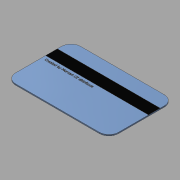
# Autodesk Inventor part: card
Saved by Autodesk Inventor 2014 SP2 (Build 180246200, 246)
## iProperties
Created: 2016-01-21
Part Number: card
Material: ABS plast
Document SubType Name: Modeling
Designer: Mervart
Mass: 4.83646 g
Surface Area: 97.3494 cm^2
Volume: 4.56269 cm^3
Density: 1.06 g/cm^3
Appearance: Hladká – bílá
LastSaveDate: 21.09.2010
Hmotnost: 0
Author: Mervart
Autodesk Inventor part; units mm, degrees
(part 1 of 2)
ref_plane "YZ Plane" through (0, 0, 0) normal (1, 0, 0) x (0, 1, 0)
sketch "Náčrt4" plane through (0, 0, 0) normal (0, 0, 1) x (1, 0, 0)
  line L0 (-42.75, -27) -> (42.75, -27)
  line L1 (42.75, -27) -> (42.75, 27)
  line L2 (42.75, 27) -> (-42.75, 27)
  line L3 (-42.75, 27) -> (-42.75, -27)
  line L4 (-42.75, -27) -> (42.75, 27) construction
  line L5 (42.75, -27) -> (-42.75, 27) construction
  point P0 (0, 0)
  dimension "d0" = 85.5
  dimension "d1" = 54
  constraints: 12 end point, 2 midpoint, 2 parallel, 1 horizontal, 1 perpendicular
  measures "d0" distance of L2.end L1.end
  measures "d1" distance of L2.end L0.start
extrude "Vysunutí1" add sketch "Náčrt4" along normal blind 1
fillet "Zaoblení1" radius 8 4 edges at (42.75, -27, 0.5) (42.75, 27, 0.5) (-42.75, 27, 0.5) (-42.75, -27, 0.5)
sketch "Náčrt5" plane through (0, 0, 1) normal (0, 0, 1) x (1, 0, 0)
  arc A0 (-42.75, -19) -> (-34.75, -27) centre (-34.75, -19) ccw construction
  line L0 (-34.75, -27) -> (34.75, -27) construction
  arc A1 (34.75, -27) -> (42.75, -19) centre (34.75, -19) ccw construction
  line L1 (42.75, -19) -> (42.75, 19) construction
  arc A2 (42.75, 19) -> (34.75, 27) centre (34.75, 19) ccw construction
  line L2 (34.75, 27) -> (-34.75, 27) construction
  arc A3 (-34.75, 27) -> (-42.75, 19) centre (-34.75, 19) ccw construction
  line L3 (-42.75, 19) -> (-42.75, -19) construction
  line L4 (42.75, 15.5948) -> (-42.75, 15.5948)
  line L5 (42.75, 5.8734) -> (-42.75, 5.8734)
  line L6 (-42.75, 5.8734) -> (-42.75, 15.5948)
  line L7 (42.75, 5.8734) -> (42.75, 15.5948)
  point P0 (0, 0)
  constraints: 8 end point, 4 point on line, 2 collinear, 2 perpendicular
ref_plane "Pracovní rovina1" through (42.75, 5.8734, 1) normal (0, 1, 0) x (-1, 0, 0)
ref_plane "Pracovní rovina2" through (42.75, 15.5948, 1) normal (0, 1, 0) x (-1, 0, 0)
split body "Rozdělit1" result two bodies by plane through (42.75, 15.5948, 1) normal (0, 1, 0) first body at (-11.5833, 19.3965, 0.5)
split body "Rozdělit2" result two bodies by plane through (42.75, 5.8734, 1) normal (0, 1, 0) bodies 3 first body at (-14.25, 12.3543, 0.5)
sketch "Náčrt6" plane through (0, 0, 1) normal (0, 0, 1) x (1, 0, 0)
  line L0 (-40.2387, 4.1503) -> (29.6053, 4.1503) construction
  line L1 (29.6053, 4.1503) -> (29.6053, -0.4729) construction
  line L2 (29.6053, -0.4729) -> (-40.2387, -0.4729) construction
  line L3 (-40.2387, -0.4729) -> (-40.2387, 4.1503) construction
  spline S0 degree 2 poles (-39.2549, 2.0255) (-39.4494, 2.0255) (-39.7784, 2.1567) (-39.8983, 2.288) knots 0 0 0 1 2 2 2
  spline S1 degree 2 poles (-39.8983, 2.288) (-40.0183, 2.4177) (-40.1496, 2.8067) (-40.1496, 3.0595) knots 0 0 0 1 2 2 2
  spline S2 degree 2 poles (-40.1496, 3.0595) (-40.1496, 3.3107) (-40.0215, 3.6835) (-39.9, 3.8213) knots 0 0 0 1 2 2 2
  spline S3 degree 2 poles (-39.9, 3.8213) (-39.78, 3.9558) (-39.4526, 4.0968) (-39.2501, 4.0968) knots 0 0 0 1 2 2 2
  spline S4 degree 2 poles (-39.2501, 4.0968) (-39.1496, 4.0968) (-38.9729, 4.0676) (-38.8983, 4.0449) knots 0 0 0 1 2 2 2
  spline S5 degree 2 poles (-38.8983, 4.0449) (-38.8335, 4.0238) (-38.699, 3.9639) (-38.6325, 3.9282) knots 0 0 0 1 2 2 2
  line L4 (-38.6325, 3.9282) -> (-38.6325, 3.6073)
  line L5 (-38.6325, 3.6073) -> (-38.6536, 3.6073)
  spline S6 degree 2 poles (-38.6536, 3.6073) (-38.6893, 3.6397) (-38.7995, 3.7305) (-38.8789, 3.7742) knots 0 0 0 1 2 2 2
  spline S7 degree 2 poles (-38.8789, 3.7742) (-38.9551, 3.8164) (-39.135, 3.8699) (-39.2517, 3.8699) knots 0 0 0 1 2 2 2
  spline S8 degree 2 poles (-39.2517, 3.8699) (-39.3797, 3.8699) (-39.6082, 3.7645) (-39.6941, 3.664) knots 0 0 0 1 2 2 2
  spline S9 degree 2 poles (-39.6941, 3.664) (-39.7784, 3.5619) (-39.8724, 3.2524) (-39.8724, 3.0595) knots 0 0 0 1 2 2 2
  spline S10 degree 2 poles (-39.8724, 3.0595) (-39.8724, 2.8537) (-39.7736, 2.5571) (-39.6877, 2.455) knots 0 0 0 1 2 2 2
  spline S11 degree 2 poles (-39.6877, 2.455) (-39.6034, 2.3561) (-39.3781, 2.2556) (-39.2517, 2.2556) knots 0 0 0 1 2 2 2
  spline S12 degree 2 poles (-39.2517, 2.2556) (-39.1366, 2.2556) (-38.9405, 2.3123) (-38.8643, 2.3545) knots 0 0 0 1 2 2 2
  spline S13 degree 2 poles (-38.8643, 2.3545) (-38.7914, 2.3966) (-38.6828, 2.4841) (-38.652, 2.5149) knots 0 0 0 1 2 2 2
  line L6 (-38.652, 2.5149) -> (-38.6325, 2.5149)
  line L7 (-38.6325, 2.5149) -> (-38.6325, 2.1973)
  spline S14 degree 2 poles (-38.6325, 2.1973) (-38.699, 2.1665) (-38.8157, 2.1097) (-38.8983, 2.0838) knots 0 0 0 1 2 2 2
  spline S15 degree 2 poles (-38.8983, 2.0838) (-38.9859, 2.0546) (-39.135, 2.0255) (-39.2549, 2.0255) knots 0 0 0 1 2 2 2
  line L8 (-37.6082, 3.2913) -> (-37.6212, 3.2913)
  spline S16 degree 2 poles (-37.6212, 3.2913) (-37.6504, 3.2994) (-37.7136, 3.3026) (-37.7573, 3.3026) knots 0 0 0 1 2 2 2
  spline S17 degree 2 poles (-37.7573, 3.3026) (-37.8595, 3.3026) (-38.0604, 3.2135) (-38.1512, 3.126) knots 0 0 0 1 2 2 2
  line L9 (-38.1512, 3.126) -> (-38.1512, 2.0611)
  line L10 (-38.1512, 2.0611) -> (-38.404, 2.0611)
  line L11 (-38.404, 2.0611) -> (-38.404, 3.5619)
  line L12 (-38.404, 3.5619) -> (-38.1512, 3.5619)
  line L13 (-38.1512, 3.5619) -> (-38.1512, 3.3383)
  spline S18 degree 2 poles (-38.1512, 3.3383) (-38.0134, 3.4614) (-37.8076, 3.5619) (-37.7103, 3.5619) knots 0 0 0 1 2 2 2
  spline S19 degree 2 poles (-37.7103, 3.5619) (-37.6714, 3.5619) (-37.6325, 3.5587) (-37.6082, 3.5538) knots 0 0 0 1 2 2 2
  line L14 (-37.6082, 3.5538) -> (-37.6082, 3.2913)
  spline S20 degree 2 poles (-36.7606, 2.0271) (-37.1204, 2.0271) (-37.5159, 2.4307) (-37.5159, 2.8034) knots 0 0 0 1 2 2 2
  spline S21 degree 2 poles (-37.5159, 2.8034) (-37.5159, 3.1697) (-37.1317, 3.6041) (-36.8222, 3.6041) knots 0 0 0 1 2 2 2
  spline S22 degree 2 poles (-36.8222, 3.6041) (-36.6828, 3.6041) (-36.4672, 3.523) (-36.3878, 3.4371) knots 0 0 0 1 2 2 2
  spline S23 degree 2 poles (-36.3878, 3.4371) (-36.3068, 3.3512) (-36.2209, 3.1033) (-36.2209, 2.9234) knots 0 0 0 1 2 2 2
  line L15 (-36.2209, 2.9234) -> (-36.2209, 2.7856)
  line L16 (-36.2209, 2.7856) -> (-37.2598, 2.7856)
  spline S24 degree 2 poles (-37.2598, 2.7856) (-37.2598, 2.5247) (-36.9972, 2.2475) (-36.7638, 2.2475) knots 0 0 0 1 2 2 2
  spline S25 degree 2 poles (-36.7638, 2.2475) (-36.6812, 2.2475) (-36.5207, 2.2848) (-36.4559, 2.314) knots 0 0 0 1 2 2 2
  spline S26 degree 2 poles (-36.4559, 2.314) (-36.3878, 2.3464) (-36.2938, 2.4031) (-36.263, 2.429) knots 0 0 0 1 2 2 2
  line L17 (-36.263, 2.429) -> (-36.2484, 2.429)
  line L18 (-36.2484, 2.429) -> (-36.2484, 2.1535)
  spline S27 degree 2 poles (-36.2484, 2.1535) (-36.2922, 2.1357) (-36.4251, 2.0838) (-36.477, 2.0692) knots 0 0 0 1 2 2 2
  spline S28 degree 2 poles (-36.477, 2.0692) (-36.5499, 2.0482) (-36.6698, 2.0271) (-36.7606, 2.0271) knots 0 0 0 1 2 2 2
  spline S29 degree 2 poles (-36.4672, 2.9785) (-36.4705, 3.0806) (-36.5126, 3.2297) (-36.5531, 3.2799) knots 0 0 0 1 2 2 2
  spline S30 degree 2 poles (-36.5531, 3.2799) (-36.5969, 3.3366) (-36.7347, 3.3966) (-36.8368, 3.3966) knots 0 0 0 1 2 2 2
  spline S31 degree 2 poles (-36.8368, 3.3966) (-36.9372, 3.3966) (-37.0783, 3.3366) (-37.1366, 3.2783) knots 0 0 0 1 2 2 2
  spline S32 degree 2 poles (-37.1366, 3.2783) (-37.1933, 3.2183) (-37.2517, 3.0741) (-37.2598, 2.9785) knots 0 0 0 1 2 2 2
  line L19 (-37.2598, 2.9785) -> (-36.4672, 2.9785)
  spline S33 degree 2 poles (-35.1285, 2.22) (-35.1593, 2.1973) (-35.263, 2.1162) (-35.3116, 2.0919) knots 0 0 0 1 2 2 2
  spline S34 degree 2 poles (-35.3116, 2.0919) (-35.3781, 2.0563) (-35.5029, 2.019) (-35.6163, 2.019) knots 0 0 0 1 2 2 2
  spline S35 degree 2 poles (-35.6163, 2.019) (-35.7087, 2.019) (-35.8757, 2.0887) (-35.9389, 2.1519) knots 0 0 0 1 2 2 2
  spline S36 degree 2 poles (-35.9389, 2.1519) (-35.9988, 2.2135) (-36.0718, 2.395) (-36.0718, 2.4955) knots 0 0 0 1 2 2 2
  spline S37 degree 2 poles (-36.0718, 2.4955) (-36.0718, 2.6511) (-35.9405, 2.8715) (-35.7979, 2.9347) knots 0 0 0 1 2 2 2
  spline S38 degree 2 poles (-35.7979, 2.9347) (-35.6714, 2.9931) (-35.3278, 3.0368) (-35.1285, 3.0482) knots 0 0 0 1 2 2 2
  line L20 (-35.1285, 3.0482) -> (-35.1285, 3.0968)
  spline S39 degree 2 poles (-35.1285, 3.0968) (-35.1285, 3.1843) (-35.182, 3.2929) (-35.2306, 3.3237) knots 0 0 0 1 2 2 2
  spline S40 degree 2 poles (-35.2306, 3.3237) (-35.2792, 3.3545) (-35.4186, 3.3739) (-35.4932, 3.3739) knots 0 0 0 1 2 2 2
  spline S41 degree 2 poles (-35.4932, 3.3739) (-35.5807, 3.3739) (-35.8173, 3.3221) (-35.9356, 3.2718) knots 0 0 0 1 2 2 2
  line L21 (-35.9356, 3.2718) -> (-35.9502, 3.2718)
  line L22 (-35.9502, 3.2718) -> (-35.9502, 3.5295)
  spline S42 degree 2 poles (-35.9502, 3.5295) (-35.8805, 3.549) (-35.6196, 3.5976) (-35.4915, 3.5976) knots 0 0 0 1 2 2 2
  spline S43 degree 2 poles (-35.4915, 3.5976) (-35.336, 3.5976) (-35.1236, 3.549) (-35.0394, 3.4858) knots 0 0 0 1 2 2 2
  spline S44 degree 2 poles (-35.0394, 3.4858) (-34.9567, 3.4242) (-34.8757, 3.2281) (-34.8757, 3.0871) knots 0 0 0 1 2 2 2
  line L23 (-34.8757, 3.0871) -> (-34.8757, 2.0611)
  line L24 (-34.8757, 2.0611) -> (-35.1285, 2.0611)
  line L25 (-35.1285, 2.0611) -> (-35.1285, 2.22)
  line L26 (-35.1285, 2.4307) -> (-35.1285, 2.8472)
  spline S45 degree 2 poles (-35.1285, 2.8472) (-35.2193, 2.8391) (-35.4932, 2.8115) (-35.5791, 2.7856) knots 0 0 0 1 2 2 2
  spline S46 degree 2 poles (-35.5791, 2.7856) (-35.6795, 2.7548) (-35.8108, 2.6268) (-35.8108, 2.5133) knots 0 0 0 1 2 2 2
  spline S47 degree 2 poles (-35.8108, 2.5133) (-35.8108, 2.3837) (-35.665, 2.2524) (-35.5256, 2.2524) knots 0 0 0 1 2 2 2
  spline S48 degree 2 poles (-35.5256, 2.2524) (-35.4073, 2.2524) (-35.2128, 2.3545) (-35.1285, 2.4307) knots 0 0 0 1 2 2 2
  spline S49 degree 2 poles (-34.0669, 2.0319) (-34.2727, 2.0319) (-34.5045, 2.267) (-34.5045, 2.5214) knots 0 0 0 1 2 2 2
  line L27 (-34.5045, 2.5214) -> (-34.5045, 3.3529)
  line L28 (-34.5045, 3.3529) -> (-34.6747, 3.3529)
  line L29 (-34.6747, 3.3529) -> (-34.6747, 3.5619)
  line L30 (-34.6747, 3.5619) -> (-34.5045, 3.5619)
  line L31 (-34.5045, 3.5619) -> (-34.5045, 3.9931)
  line L32 (-34.5045, 3.9931) -> (-34.2517, 3.9931)
  line L33 (-34.2517, 3.9931) -> (-34.2517, 3.5619)
  line L34 (-34.2517, 3.5619) -> (-33.7865, 3.5619)
  line L35 (-33.7865, 3.5619) -> (-33.7865, 3.3529)
  line L36 (-33.7865, 3.3529) -> (-34.2517, 3.3529)
  line L37 (-34.2517, 3.3529) -> (-34.2517, 2.6381)
  spline S50 degree 2 poles (-34.2517, 2.6381) (-34.2517, 2.5247) (-34.2436, 2.3999) (-34.216, 2.3464) knots 0 0 0 1 2 2 2
  spline S51 degree 2 poles (-34.216, 2.3464) (-34.1933, 2.2994) (-34.0912, 2.2524) (-34.0037, 2.2524) knots 0 0 0 1 2 2 2
  spline S52 degree 2 poles (-34.0037, 2.2524) (-33.9421, 2.2524) (-33.827, 2.2896) (-33.8011, 2.301) knots 0 0 0 1 2 2 2
  line L38 (-33.8011, 2.301) -> (-33.7865, 2.301)
  line L39 (-33.7865, 2.301) -> (-33.7865, 2.0741)
  spline S53 degree 2 poles (-33.7865, 2.0741) (-33.8578, 2.0546) (-34.0037, 2.0319) (-34.0669, 2.0319) knots 0 0 0 1 2 2 2
  spline S54 degree 2 poles (-32.9486, 2.0271) (-33.3084, 2.0271) (-33.7039, 2.4307) (-33.7039, 2.8034) knots 0 0 0 1 2 2 2
  spline S55 degree 2 poles (-33.7039, 2.8034) (-33.7039, 3.1697) (-33.3197, 3.6041) (-33.0102, 3.6041) knots 0 0 0 1 2 2 2
  spline S56 degree 2 poles (-33.0102, 3.6041) (-32.8708, 3.6041) (-32.6552, 3.523) (-32.5758, 3.4371) knots 0 0 0 1 2 2 2
  spline S57 degree 2 poles (-32.5758, 3.4371) (-32.4948, 3.3512) (-32.4089, 3.1033) (-32.4089, 2.9234) knots 0 0 0 1 2 2 2
  line L40 (-32.4089, 2.9234) -> (-32.4089, 2.7856)
  line L41 (-32.4089, 2.7856) -> (-33.4478, 2.7856)
  spline S58 degree 2 poles (-33.4478, 2.7856) (-33.4478, 2.5247) (-33.1852, 2.2475) (-32.9518, 2.2475) knots 0 0 0 1 2 2 2
  spline S59 degree 2 poles (-32.9518, 2.2475) (-32.8692, 2.2475) (-32.7087, 2.2848) (-32.6439, 2.314) knots 0 0 0 1 2 2 2
  spline S60 degree 2 poles (-32.6439, 2.314) (-32.5758, 2.3464) (-32.4818, 2.4031) (-32.451, 2.429) knots 0 0 0 1 2 2 2
  line L42 (-32.451, 2.429) -> (-32.4364, 2.429)
  line L43 (-32.4364, 2.429) -> (-32.4364, 2.1535)
  spline S61 degree 2 poles (-32.4364, 2.1535) (-32.4802, 2.1357) (-32.6131, 2.0838) (-32.665, 2.0692) knots 0 0 0 1 2 2 2
  spline S62 degree 2 poles (-32.665, 2.0692) (-32.7379, 2.0482) (-32.8578, 2.0271) (-32.9486, 2.0271) knots 0 0 0 1 2 2 2
  spline S63 degree 2 poles (-32.6552, 2.9785) (-32.6585, 3.0806) (-32.7006, 3.2297) (-32.7411, 3.2799) knots 0 0 0 1 2 2 2
  spline S64 degree 2 poles (-32.7411, 3.2799) (-32.7849, 3.3366) (-32.9227, 3.3966) (-33.0248, 3.3966) knots 0 0 0 1 2 2 2
  spline S65 degree 2 poles (-33.0248, 3.3966) (-33.1253, 3.3966) (-33.2663, 3.3366) (-33.3246, 3.2783) knots 0 0 0 1 2 2 2
  spline S66 degree 2 poles (-33.3246, 3.2783) (-33.3813, 3.2183) (-33.4397, 3.0741) (-33.4478, 2.9785) knots 0 0 0 1 2 2 2
  line L44 (-33.4478, 2.9785) -> (-32.6552, 2.9785)
  line L45 (-30.9988, 2.0611) -> (-31.2517, 2.0611)
  line L46 (-31.2517, 2.0611) -> (-31.2517, 2.2135)
  spline S67 degree 2 poles (-31.2517, 2.2135) (-31.31, 2.1648) (-31.3959, 2.1) (-31.4543, 2.0725) knots 0 0 0 1 2 2 2
  spline S68 degree 2 poles (-31.4543, 2.0725) (-31.5077, 2.0465) (-31.6228, 2.019) (-31.699, 2.019) knots 0 0 0 1 2 2 2
  spline S69 degree 2 poles (-31.699, 2.019) (-31.8222, 2.019) (-32.0296, 2.1211) (-32.1026, 2.22) knots 0 0 0 1 2 2 2
  spline S70 degree 2 poles (-32.1026, 2.22) (-32.1755, 2.3188) (-32.2565, 2.6106) (-32.2565, 2.8002) knots 0 0 0 1 2 2 2
  spline S71 degree 2 poles (-32.2565, 2.8002) (-32.2565, 2.9979) (-32.1544, 3.2864) (-32.0653, 3.395) knots 0 0 0 1 2 2 2
  spline S72 degree 2 poles (-32.0653, 3.395) (-31.9826, 3.4922) (-31.7509, 3.6041) (-31.6228, 3.6041) knots 0 0 0 1 2 2 2
  spline S73 degree 2 poles (-31.6228, 3.6041) (-31.511, 3.6041) (-31.3441, 3.5538) (-31.2517, 3.502) knots 0 0 0 1 2 2 2
  line L47 (-31.2517, 3.502) -> (-31.2517, 4.1503)
  line L48 (-31.2517, 4.1503) -> (-30.9988, 4.1503)
  line L49 (-30.9988, 4.1503) -> (-30.9988, 2.0611)
  line L50 (-31.2517, 2.4258) -> (-31.2517, 3.2929)
  spline S74 degree 2 poles (-31.2517, 3.2929) (-31.3457, 3.3383) (-31.4948, 3.3723) (-31.5807, 3.3723) knots 0 0 0 1 2 2 2
  spline S75 degree 2 poles (-31.5807, 3.3723) (-31.7752, 3.3723) (-31.9956, 3.0806) (-31.9956, 2.805) knots 0 0 0 1 2 2 2
  spline S76 degree 2 poles (-31.9956, 2.805) (-31.9956, 2.5392) (-31.827, 2.2589) (-31.6407, 2.2589) knots 0 0 0 1 2 2 2
  spline S77 degree 2 poles (-31.6407, 2.2589) (-31.5418, 2.2589) (-31.3408, 2.3496) (-31.2517, 2.4258) knots 0 0 0 1 2 2 2
  spline S78 degree 2 poles (-28.5159, 2.8358) (-28.5159, 2.4679) (-28.8724, 2.019) (-29.1415, 2.019) knots 0 0 0 1 2 2 2
  spline S79 degree 2 poles (-29.1415, 2.019) (-29.263, 2.019) (-29.4364, 2.0789) (-29.5207, 2.1308) knots 0 0 0 1 2 2 2
  line L51 (-29.5207, 2.1308) -> (-29.5369, 2.0611)
  line L52 (-29.5369, 2.0611) -> (-29.7736, 2.0611)
  line L53 (-29.7736, 2.0611) -> (-29.7736, 4.1503)
  line L54 (-29.7736, 4.1503) -> (-29.5207, 4.1503)
  line L55 (-29.5207, 4.1503) -> (-29.5207, 3.4047)
  spline S80 degree 2 poles (-29.5207, 3.4047) (-29.4251, 3.4906) (-29.203, 3.6041) (-29.062, 3.6041) knots 0 0 0 1 2 2 2
  spline S81 degree 2 poles (-29.062, 3.6041) (-28.8076, 3.6041) (-28.5159, 3.1973) (-28.5159, 2.8358) knots 0 0 0 1 2 2 2
  spline S82 degree 2 poles (-28.7768, 2.8164) (-28.7768, 3.0854) (-28.9405, 3.3642) (-29.122, 3.3642) knots 0 0 0 1 2 2 2
  spline S83 degree 2 poles (-29.122, 3.3642) (-29.2241, 3.3642) (-29.4348, 3.267) (-29.5207, 3.1924) knots 0 0 0 1 2 2 2
  line L56 (-29.5207, 3.1924) -> (-29.5207, 2.3318)
  spline S84 degree 2 poles (-29.5207, 2.3318) (-29.4251, 2.2848) (-29.2776, 2.2459) (-29.1901, 2.2459) knots 0 0 0 1 2 2 2
  spline S85 degree 2 poles (-29.1901, 2.2459) (-28.9972, 2.2459) (-28.7768, 2.5198) (-28.7768, 2.8164) knots 0 0 0 1 2 2 2
  line L57 (-27.075, 3.5619) -> (-27.8821, 1.5084)
  line L58 (-27.8821, 1.5084) -> (-28.1528, 1.5084)
  line L59 (-28.1528, 1.5084) -> (-27.8838, 2.1341)
  line L60 (-27.8838, 2.1341) -> (-28.4283, 3.5619)
  line L61 (-28.4283, 3.5619) -> (-28.156, 3.5619)
  line L62 (-28.156, 3.5619) -> (-27.746, 2.4501)
  line L63 (-27.746, 2.4501) -> (-27.3376, 3.5619)
  line L64 (-27.3376, 3.5619) -> (-27.075, 3.5619)
  line L65 (-24.2906, 2.0611) -> (-24.5564, 2.0611)
  line L66 (-24.5564, 2.0611) -> (-24.5564, 3.784)
  line L67 (-24.5564, 3.784) -> (-25.0783, 2.6122)
  line L68 (-25.0783, 2.6122) -> (-25.2403, 2.6122)
  line L69 (-25.2403, 2.6122) -> (-25.7573, 3.784)
  line L70 (-25.7573, 3.784) -> (-25.7573, 2.0611)
  line L71 (-25.7573, 2.0611) -> (-26.0053, 2.0611)
  line L72 (-26.0053, 2.0611) -> (-26.0053, 4.0611)
  line L73 (-26.0053, 4.0611) -> (-25.6423, 4.0611)
  line L74 (-25.6423, 4.0611) -> (-25.1431, 2.9477)
  line L75 (-25.1431, 2.9477) -> (-24.6601, 4.0611)
  line L76 (-24.6601, 4.0611) -> (-24.2906, 4.0611)
  line L77 (-24.2906, 4.0611) -> (-24.2906, 2.0611)
  spline S86 degree 2 poles (-23.2533, 2.0271) (-23.6131, 2.0271) (-24.0086, 2.4307) (-24.0086, 2.8034) knots 0 0 0 1 2 2 2
  spline S87 degree 2 poles (-24.0086, 2.8034) (-24.0086, 3.1697) (-23.6244, 3.6041) (-23.3149, 3.6041) knots 0 0 0 1 2 2 2
  spline S88 degree 2 poles (-23.3149, 3.6041) (-23.1755, 3.6041) (-22.9599, 3.523) (-22.8805, 3.4371) knots 0 0 0 1 2 2 2
  spline S89 degree 2 poles (-22.8805, 3.4371) (-22.7995, 3.3512) (-22.7136, 3.1033) (-22.7136, 2.9234) knots 0 0 0 1 2 2 2
  line L78 (-22.7136, 2.9234) -> (-22.7136, 2.7856)
  line L79 (-22.7136, 2.7856) -> (-23.7525, 2.7856)
  spline S90 degree 2 poles (-23.7525, 2.7856) (-23.7525, 2.5247) (-23.4899, 2.2475) (-23.2565, 2.2475) knots 0 0 0 1 2 2 2
  spline S91 degree 2 poles (-23.2565, 2.2475) (-23.1739, 2.2475) (-23.0134, 2.2848) (-22.9486, 2.314) knots 0 0 0 1 2 2 2
  spline S92 degree 2 poles (-22.9486, 2.314) (-22.8805, 2.3464) (-22.7865, 2.4031) (-22.7557, 2.429) knots 0 0 0 1 2 2 2
  line L80 (-22.7557, 2.429) -> (-22.7411, 2.429)
  line L81 (-22.7411, 2.429) -> (-22.7411, 2.1535)
  spline S93 degree 2 poles (-22.7411, 2.1535) (-22.7849, 2.1357) (-22.9178, 2.0838) (-22.9697, 2.0692) knots 0 0 0 1 2 2 2
  spline S94 degree 2 poles (-22.9697, 2.0692) (-23.0426, 2.0482) (-23.1625, 2.0271) (-23.2533, 2.0271) knots 0 0 0 1 2 2 2
  spline S95 degree 2 poles (-22.9599, 2.9785) (-22.9632, 3.0806) (-23.0053, 3.2297) (-23.0458, 3.2799) knots 0 0 0 1 2 2 2
  spline S96 degree 2 poles (-23.0458, 3.2799) (-23.0896, 3.3366) (-23.2274, 3.3966) (-23.3295, 3.3966) knots 0 0 0 1 2 2 2
  spline S97 degree 2 poles (-23.3295, 3.3966) (-23.43, 3.3966) (-23.571, 3.3366) (-23.6293, 3.2783) knots 0 0 0 1 2 2 2
  spline S98 degree 2 poles (-23.6293, 3.2783) (-23.686, 3.2183) (-23.7444, 3.0741) (-23.7525, 2.9785) knots 0 0 0 1 2 2 2
  line L82 (-23.7525, 2.9785) -> (-22.9599, 2.9785)
  line L83 (-21.6617, 3.2913) -> (-21.6747, 3.2913)
  spline S99 degree 2 poles (-21.6747, 3.2913) (-21.7039, 3.2994) (-21.7671, 3.3026) (-21.8108, 3.3026) knots 0 0 0 1 2 2 2
  spline S100 degree 2 poles (-21.8108, 3.3026) (-21.9129, 3.3026) (-22.1139, 3.2135) (-22.2047, 3.126) knots 0 0 0 1 2 2 2
  line L84 (-22.2047, 3.126) -> (-22.2047, 2.0611)
  line L85 (-22.2047, 2.0611) -> (-22.4575, 2.0611)
  line L86 (-22.4575, 2.0611) -> (-22.4575, 3.5619)
  line L87 (-22.4575, 3.5619) -> (-22.2047, 3.5619)
  line L88 (-22.2047, 3.5619) -> (-22.2047, 3.3383)
  spline S101 degree 2 poles (-22.2047, 3.3383) (-22.0669, 3.4614) (-21.8611, 3.5619) (-21.7638, 3.5619) knots 0 0 0 1 2 2 2
  spline S102 degree 2 poles (-21.7638, 3.5619) (-21.7249, 3.5619) (-21.686, 3.5587) (-21.6617, 3.5538) knots 0 0 0 1 2 2 2
  line L89 (-21.6617, 3.5538) -> (-21.6617, 3.2913)
  line L90 (-20.2873, 3.5619) -> (-20.853, 2.0611)
  line L91 (-20.853, 2.0611) -> (-21.0799, 2.0611)
  line L92 (-21.0799, 2.0611) -> (-21.6406, 3.5619)
  line L93 (-21.6406, 3.5619) -> (-21.3667, 3.5619)
  line L94 (-21.3667, 3.5619) -> (-20.9567, 2.4063)
  line L95 (-20.9567, 2.4063) -> (-20.5499, 3.5619)
  line L96 (-20.5499, 3.5619) -> (-20.2873, 3.5619)
  spline S103 degree 2 poles (-19.2598, 2.22) (-19.2906, 2.1973) (-19.3943, 2.1162) (-19.4429, 2.0919) knots 0 0 0 1 2 2 2
  spline S104 degree 2 poles (-19.4429, 2.0919) (-19.5094, 2.0563) (-19.6342, 2.019) (-19.7476, 2.019) knots 0 0 0 1 2 2 2
  spline S105 degree 2 poles (-19.7476, 2.019) (-19.84, 2.019) (-20.0069, 2.0887) (-20.0701, 2.1519) knots 0 0 0 1 2 2 2
  spline S106 degree 2 poles (-20.0701, 2.1519) (-20.1301, 2.2135) (-20.203, 2.395) (-20.203, 2.4955) knots 0 0 0 1 2 2 2
  spline S107 degree 2 poles (-20.203, 2.4955) (-20.203, 2.6511) (-20.0718, 2.8715) (-19.9291, 2.9347) knots 0 0 0 1 2 2 2
  spline S108 degree 2 poles (-19.9291, 2.9347) (-19.8027, 2.9931) (-19.4591, 3.0368) (-19.2598, 3.0482) knots 0 0 0 1 2 2 2
  line L97 (-19.2598, 3.0482) -> (-19.2598, 3.0968)
  spline S109 degree 2 poles (-19.2598, 3.0968) (-19.2598, 3.1843) (-19.3133, 3.2929) (-19.3619, 3.3237) knots 0 0 0 1 2 2 2
  spline S110 degree 2 poles (-19.3619, 3.3237) (-19.4105, 3.3545) (-19.5499, 3.3739) (-19.6244, 3.3739) knots 0 0 0 1 2 2 2
  spline S111 degree 2 poles (-19.6244, 3.3739) (-19.712, 3.3739) (-19.9486, 3.3221) (-20.0669, 3.2718) knots 0 0 0 1 2 2 2
  line L98 (-20.0669, 3.2718) -> (-20.0815, 3.2718)
  line L99 (-20.0815, 3.2718) -> (-20.0815, 3.5295)
  spline S112 degree 2 poles (-20.0815, 3.5295) (-20.0118, 3.549) (-19.7509, 3.5976) (-19.6228, 3.5976) knots 0 0 0 1 2 2 2
  spline S113 degree 2 poles (-19.6228, 3.5976) (-19.4672, 3.5976) (-19.2549, 3.549) (-19.1706, 3.4858) knots 0 0 0 1 2 2 2
  spline S114 degree 2 poles (-19.1706, 3.4858) (-19.088, 3.4242) (-19.0069, 3.2281) (-19.0069, 3.0871) knots 0 0 0 1 2 2 2
  line L100 (-19.0069, 3.0871) -> (-19.0069, 2.0611)
  line L101 (-19.0069, 2.0611) -> (-19.2598, 2.0611)
  line L102 (-19.2598, 2.0611) -> (-19.2598, 2.22)
  line L103 (-19.2598, 2.4307) -> (-19.2598, 2.8472)
  spline S115 degree 2 poles (-19.2598, 2.8472) (-19.3505, 2.8391) (-19.6244, 2.8115) (-19.7103, 2.7856) knots 0 0 0 1 2 2 2
  spline S116 degree 2 poles (-19.7103, 2.7856) (-19.8108, 2.7548) (-19.9421, 2.6268) (-19.9421, 2.5133) knots 0 0 0 1 2 2 2
  spline S117 degree 2 poles (-19.9421, 2.5133) (-19.9421, 2.3837) (-19.7962, 2.2524) (-19.6569, 2.2524) knots 0 0 0 1 2 2 2
  spline S118 degree 2 poles (-19.6569, 2.2524) (-19.5385, 2.2524) (-19.3441, 2.3545) (-19.2598, 2.4307) knots 0 0 0 1 2 2 2
  line L104 (-17.8562, 3.2913) -> (-17.8692, 3.2913)
  spline S119 degree 2 poles (-17.8692, 3.2913) (-17.8983, 3.2994) (-17.9616, 3.3026) (-18.0053, 3.3026) knots 0 0 0 1 2 2 2
  spline S120 degree 2 poles (-18.0053, 3.3026) (-18.1074, 3.3026) (-18.3084, 3.2135) (-18.3992, 3.126) knots 0 0 0 1 2 2 2
  line L105 (-18.3992, 3.126) -> (-18.3992, 2.0611)
  line L106 (-18.3992, 2.0611) -> (-18.652, 2.0611)
  line L107 (-18.652, 2.0611) -> (-18.652, 3.5619)
  line L108 (-18.652, 3.5619) -> (-18.3992, 3.5619)
  line L109 (-18.3992, 3.5619) -> (-18.3992, 3.3383)
  spline S121 degree 2 poles (-18.3992, 3.3383) (-18.2614, 3.4614) (-18.0556, 3.5619) (-17.9583, 3.5619) knots 0 0 0 1 2 2 2
  spline S122 degree 2 poles (-17.9583, 3.5619) (-17.9194, 3.5619) (-17.8805, 3.5587) (-17.8562, 3.5538) knots 0 0 0 1 2 2 2
  line L110 (-17.8562, 3.5538) -> (-17.8562, 3.2913)
  spline S123 degree 2 poles (-17.2063, 2.0319) (-17.4121, 2.0319) (-17.6439, 2.267) (-17.6439, 2.5214) knots 0 0 0 1 2 2 2
  line L111 (-17.6439, 2.5214) -> (-17.6439, 3.3529)
  line L112 (-17.6439, 3.3529) -> (-17.8141, 3.3529)
  line L113 (-17.8141, 3.3529) -> (-17.8141, 3.5619)
  line L114 (-17.8141, 3.5619) -> (-17.6439, 3.5619)
  line L115 (-17.6439, 3.5619) -> (-17.6439, 3.9931)
  line L116 (-17.6439, 3.9931) -> (-17.3911, 3.9931)
  line L117 (-17.3911, 3.9931) -> (-17.3911, 3.5619)
  line L118 (-17.3911, 3.5619) -> (-16.9259, 3.5619)
  line L119 (-16.9259, 3.5619) -> (-16.9259, 3.3529)
  line L120 (-16.9259, 3.3529) -> (-17.3911, 3.3529)
  line L121 (-17.3911, 3.3529) -> (-17.3911, 2.6381)
  spline S124 degree 2 poles (-17.3911, 2.6381) (-17.3911, 2.5247) (-17.383, 2.3999) (-17.3554, 2.3464) knots 0 0 0 1 2 2 2
  spline S125 degree 2 poles (-17.3554, 2.3464) (-17.3327, 2.2994) (-17.2306, 2.2524) (-17.1431, 2.2524) knots 0 0 0 1 2 2 2
  spline S126 degree 2 poles (-17.1431, 2.2524) (-17.0815, 2.2524) (-16.9664, 2.2896) (-16.9405, 2.301) knots 0 0 0 1 2 2 2
  line L122 (-16.9405, 2.301) -> (-16.9259, 2.301)
  line L123 (-16.9259, 2.301) -> (-16.9259, 2.0741)
  spline S127 degree 2 poles (-16.9259, 2.0741) (-16.9972, 2.0546) (-17.1431, 2.0319) (-17.2063, 2.0319) knots 0 0 0 1 2 2 2
  spline S128 degree 2 poles (-15.0799, 2.0255) (-15.2744, 2.0255) (-15.6034, 2.1567) (-15.7233, 2.288) knots 0 0 0 1 2 2 2
  spline S129 degree 2 poles (-15.7233, 2.288) (-15.8432, 2.4177) (-15.9745, 2.8067) (-15.9745, 3.0595) knots 0 0 0 1 2 2 2
  spline S130 degree 2 poles (-15.9745, 3.0595) (-15.9745, 3.3107) (-15.8465, 3.6835) (-15.7249, 3.8213) knots 0 0 0 1 2 2 2
  spline S131 degree 2 poles (-15.7249, 3.8213) (-15.605, 3.9558) (-15.2776, 4.0968) (-15.075, 4.0968) knots 0 0 0 1 2 2 2
  spline S132 degree 2 poles (-15.075, 4.0968) (-14.9745, 4.0968) (-14.7979, 4.0676) (-14.7233, 4.0449) knots 0 0 0 1 2 2 2
  spline S133 degree 2 poles (-14.7233, 4.0449) (-14.6585, 4.0238) (-14.524, 3.9639) (-14.4575, 3.9282) knots 0 0 0 1 2 2 2
  line L124 (-14.4575, 3.9282) -> (-14.4575, 3.6073)
  line L125 (-14.4575, 3.6073) -> (-14.4786, 3.6073)
  spline S134 degree 2 poles (-14.4786, 3.6073) (-14.5142, 3.6397) (-14.6244, 3.7305) (-14.7039, 3.7742) knots 0 0 0 1 2 2 2
  spline S135 degree 2 poles (-14.7039, 3.7742) (-14.78, 3.8164) (-14.9599, 3.8699) (-15.0766, 3.8699) knots 0 0 0 1 2 2 2
  spline S136 degree 2 poles (-15.0766, 3.8699) (-15.2047, 3.8699) (-15.4332, 3.7645) (-15.5191, 3.664) knots 0 0 0 1 2 2 2
  spline S137 degree 2 poles (-15.5191, 3.664) (-15.6034, 3.5619) (-15.6974, 3.2524) (-15.6974, 3.0595) knots 0 0 0 1 2 2 2
  spline S138 degree 2 poles (-15.6974, 3.0595) (-15.6974, 2.8537) (-15.5985, 2.5571) (-15.5126, 2.455) knots 0 0 0 1 2 2 2
  spline S139 degree 2 poles (-15.5126, 2.455) (-15.4283, 2.3561) (-15.203, 2.2556) (-15.0766, 2.2556) knots 0 0 0 1 2 2 2
  spline S140 degree 2 poles (-15.0766, 2.2556) (-14.9616, 2.2556) (-14.7654, 2.3123) (-14.6893, 2.3545) knots 0 0 0 1 2 2 2
  spline S141 degree 2 poles (-14.6893, 2.3545) (-14.6163, 2.3966) (-14.5077, 2.4841) (-14.477, 2.5149) knots 0 0 0 1 2 2 2
  line L126 (-14.477, 2.5149) -> (-14.4575, 2.5149)
  line L127 (-14.4575, 2.5149) -> (-14.4575, 2.1973)
  spline S142 degree 2 poles (-14.4575, 2.1973) (-14.524, 2.1665) (-14.6406, 2.1097) (-14.7233, 2.0838) knots 0 0 0 1 2 2 2
  spline S143 degree 2 poles (-14.7233, 2.0838) (-14.8108, 2.0546) (-14.9599, 2.0255) (-15.0799, 2.0255) knots 0 0 0 1 2 2 2
  line L128 (-12.934, 2.0611) -> (-14.3311, 2.0611)
  line L129 (-14.3311, 2.0611) -> (-14.3311, 2.3091)
  line L130 (-14.3311, 2.3091) -> (-13.2614, 3.8245)
  line L131 (-13.2614, 3.8245) -> (-14.2825, 3.8245)
  line L132 (-14.2825, 3.8245) -> (-14.2825, 4.0611)
  line L133 (-14.2825, 4.0611) -> (-12.9616, 4.0611)
  line L134 (-12.9616, 4.0611) -> (-12.9616, 3.8213)
  line L135 (-12.9616, 3.8213) -> (-14.0426, 2.2978)
  line L136 (-14.0426, 2.2978) -> (-12.934, 2.2978)
  line L137 (-12.934, 2.2978) -> (-12.934, 2.0611)
  line L138 (-10.6779, 2.0611) -> (-10.9308, 2.0611)
  line L139 (-10.9308, 2.0611) -> (-10.9308, 2.2135)
  spline S144 degree 2 poles (-10.9308, 2.2135) (-10.9891, 2.1648) (-11.075, 2.1) (-11.1334, 2.0725) knots 0 0 0 1 2 2 2
  spline S145 degree 2 poles (-11.1334, 2.0725) (-11.1868, 2.0465) (-11.3019, 2.019) (-11.3781, 2.019) knots 0 0 0 1 2 2 2
  spline S146 degree 2 poles (-11.3781, 2.019) (-11.5013, 2.019) (-11.7087, 2.1211) (-11.7817, 2.22) knots 0 0 0 1 2 2 2
  spline S147 degree 2 poles (-11.7817, 2.22) (-11.8546, 2.3188) (-11.9356, 2.6106) (-11.9356, 2.8002) knots 0 0 0 1 2 2 2
  spline S148 degree 2 poles (-11.9356, 2.8002) (-11.9356, 2.9979) (-11.8335, 3.2864) (-11.7444, 3.395) knots 0 0 0 1 2 2 2
  spline S149 degree 2 poles (-11.7444, 3.395) (-11.6617, 3.4922) (-11.43, 3.6041) (-11.3019, 3.6041) knots 0 0 0 1 2 2 2
  spline S150 degree 2 poles (-11.3019, 3.6041) (-11.1901, 3.6041) (-11.0231, 3.5538) (-10.9308, 3.502) knots 0 0 0 1 2 2 2
  line L140 (-10.9308, 3.502) -> (-10.9308, 4.1503)
  line L141 (-10.9308, 4.1503) -> (-10.6779, 4.1503)
  line L142 (-10.6779, 4.1503) -> (-10.6779, 2.0611)
  line L143 (-10.9308, 2.4258) -> (-10.9308, 3.2929)
  spline S151 degree 2 poles (-10.9308, 3.2929) (-11.0248, 3.3383) (-11.1739, 3.3723) (-11.2598, 3.3723) knots 0 0 0 1 2 2 2
  spline S152 degree 2 poles (-11.2598, 3.3723) (-11.4543, 3.3723) (-11.6747, 3.0806) (-11.6747, 2.805) knots 0 0 0 1 2 2 2
  spline S153 degree 2 poles (-11.6747, 2.805) (-11.6747, 2.5392) (-11.5061, 2.2589) (-11.3197, 2.2589) knots 0 0 0 1 2 2 2
  spline S154 degree 2 poles (-11.3197, 2.2589) (-11.2209, 2.2589) (-11.0199, 2.3496) (-10.9308, 2.4258) knots 0 0 0 1 2 2 2
  line L144 (-10.0539, 2.0611) -> (-10.3068, 2.0611)
  line L145 (-10.3068, 2.0611) -> (-10.3068, 3.5619)
  line L146 (-10.3068, 3.5619) -> (-10.0539, 3.5619)
  line L147 (-10.0539, 3.5619) -> (-10.0539, 2.0611)
  line L148 (-10.0361, 3.8115) -> (-10.323, 3.8115)
  line L149 (-10.323, 3.8115) -> (-10.323, 4.0741)
  line L150 (-10.323, 4.0741) -> (-10.0361, 4.0741)
  line L151 (-10.0361, 4.0741) -> (-10.0361, 3.8115)
  spline S155 degree 2 poles (-9.2776, 2.0255) (-9.4283, 2.0255) (-9.6893, 2.1065) (-9.7752, 2.1519) knots 0 0 0 1 2 2 2
  line L152 (-9.7752, 2.1519) -> (-9.7752, 2.4355)
  line L153 (-9.7752, 2.4355) -> (-9.7622, 2.4355)
  spline S156 degree 2 poles (-9.7622, 2.4355) (-9.7298, 2.4096) (-9.6423, 2.348) (-9.5693, 2.314) knots 0 0 0 1 2 2 2
  spline S157 degree 2 poles (-9.5693, 2.314) (-9.5061, 2.2832) (-9.3505, 2.2378) (-9.2679, 2.2378) knots 0 0 0 1 2 2 2
  spline S158 degree 2 poles (-9.2679, 2.2378) (-9.2079, 2.2378) (-9.0701, 2.2653) (-9.0377, 2.288) knots 0 0 0 1 2 2 2
  spline S159 degree 2 poles (-9.0377, 2.288) (-8.9907, 2.3188) (-8.9486, 2.3885) (-8.9486, 2.4598) knots 0 0 0 1 2 2 2
  spline S160 degree 2 poles (-8.9486, 2.4598) (-8.9486, 2.549) (-9.0458, 2.6413) (-9.1706, 2.6721) knots 0 0 0 1 2 2 2
  spline S161 degree 2 poles (-9.1706, 2.6721) (-9.2193, 2.6835) (-9.3748, 2.7159) (-9.4413, 2.7337) knots 0 0 0 1 2 2 2
  spline S162 degree 2 poles (-9.4413, 2.7337) (-9.6131, 2.784) (-9.7687, 2.9914) (-9.7687, 3.1389) knots 0 0 0 1 2 2 2
  spline S163 degree 2 poles (-9.7687, 3.1389) (-9.7687, 3.3431) (-9.4624, 3.5976) (-9.2095, 3.5976) knots 0 0 0 1 2 2 2
  spline S164 degree 2 poles (-9.2095, 3.5976) (-9.0847, 3.5976) (-8.8319, 3.536) (-8.746, 3.489) knots 0 0 0 1 2 2 2
  line L154 (-8.746, 3.489) -> (-8.746, 3.2183)
  line L155 (-8.746, 3.2183) -> (-8.759, 3.2183)
  spline S165 degree 2 poles (-8.759, 3.2183) (-8.8562, 3.2961) (-9.0928, 3.3853) (-9.2144, 3.3853) knots 0 0 0 1 2 2 2
  spline S166 degree 2 poles (-9.2144, 3.3853) (-9.3392, 3.3853) (-9.511, 3.2799) (-9.511, 3.1746) knots 0 0 0 1 2 2 2
  spline S167 degree 2 poles (-9.511, 3.1746) (-9.511, 3.0789) (-9.4089, 2.9866) (-9.2954, 2.9574) knots 0 0 0 1 2 2 2
  spline S168 degree 2 poles (-9.2954, 2.9574) (-9.2403, 2.9428) (-9.1009, 2.9136) (-9.0248, 2.8958) knots 0 0 0 1 2 2 2
  spline S169 degree 2 poles (-9.0248, 2.8958) (-8.8595, 2.8537) (-8.6909, 2.6608) (-8.6909, 2.4939) knots 0 0 0 1 2 2 2
  spline S170 degree 2 poles (-8.6909, 2.4939) (-8.6909, 2.3966) (-8.7671, 2.2248) (-8.8416, 2.1616) knots 0 0 0 1 2 2 2
  spline S171 degree 2 poles (-8.8416, 2.1616) (-8.921, 2.0952) (-9.1236, 2.0255) (-9.2776, 2.0255) knots 0 0 0 1 2 2 2
  spline S172 degree 2 poles (-8.0021, 2.0319) (-8.2079, 2.0319) (-8.4397, 2.267) (-8.4397, 2.5214) knots 0 0 0 1 2 2 2
  line L156 (-8.4397, 2.5214) -> (-8.4397, 3.3529)
  line L157 (-8.4397, 3.3529) -> (-8.6099, 3.3529)
  line L158 (-8.6099, 3.3529) -> (-8.6099, 3.5619)
  line L159 (-8.6099, 3.5619) -> (-8.4397, 3.5619)
  line L160 (-8.4397, 3.5619) -> (-8.4397, 3.9931)
  line L161 (-8.4397, 3.9931) -> (-8.1868, 3.9931)
  line L162 (-8.1868, 3.9931) -> (-8.1868, 3.5619)
  line L163 (-8.1868, 3.5619) -> (-7.7217, 3.5619)
  line L164 (-7.7217, 3.5619) -> (-7.7217, 3.3529)
  line L165 (-7.7217, 3.3529) -> (-8.1868, 3.3529)
  line L166 (-8.1868, 3.3529) -> (-8.1868, 2.6381)
  spline S173 degree 2 poles (-8.1868, 2.6381) (-8.1868, 2.5247) (-8.1787, 2.3999) (-8.1512, 2.3464) knots 0 0 0 1 2 2 2
  spline S174 degree 2 poles (-8.1512, 2.3464) (-8.1285, 2.2994) (-8.0264, 2.2524) (-7.9389, 2.2524) knots 0 0 0 1 2 2 2
  spline S175 degree 2 poles (-7.9389, 2.2524) (-7.8773, 2.2524) (-7.7622, 2.2896) (-7.7363, 2.301) knots 0 0 0 1 2 2 2
  line L167 (-7.7363, 2.301) -> (-7.7217, 2.301)
  line L168 (-7.7217, 2.301) -> (-7.7217, 2.0741)
  spline S176 degree 2 poles (-7.7217, 2.0741) (-7.793, 2.0546) (-7.9389, 2.0319) (-8.0021, 2.0319) knots 0 0 0 1 2 2 2
  line L169 (-6.7395, 3.2913) -> (-6.7525, 3.2913)
  spline S177 degree 2 poles (-6.7525, 3.2913) (-6.7817, 3.2994) (-6.8449, 3.3026) (-6.8886, 3.3026) knots 0 0 0 1 2 2 2
  spline S178 degree 2 poles (-6.8886, 3.3026) (-6.9907, 3.3026) (-7.1917, 3.2135) (-7.2825, 3.126) knots 0 0 0 1 2 2 2
  line L170 (-7.2825, 3.126) -> (-7.2825, 2.0611)
  line L171 (-7.2825, 2.0611) -> (-7.5353, 2.0611)
  line L172 (-7.5353, 2.0611) -> (-7.5353, 3.5619)
  line L173 (-7.5353, 3.5619) -> (-7.2825, 3.5619)
  line L174 (-7.2825, 3.5619) -> (-7.2825, 3.3383)
  spline S179 degree 2 poles (-7.2825, 3.3383) (-7.1447, 3.4614) (-6.9389, 3.5619) (-6.8416, 3.5619) knots 0 0 0 1 2 2 2
  spline S180 degree 2 poles (-6.8416, 3.5619) (-6.8027, 3.5619) (-6.7638, 3.5587) (-6.7395, 3.5538) knots 0 0 0 1 2 2 2
  line L175 (-6.7395, 3.5538) -> (-6.7395, 3.2913)
  line L176 (-6.2857, 2.0611) -> (-6.5385, 2.0611)
  line L177 (-6.5385, 2.0611) -> (-6.5385, 3.5619)
  line L178 (-6.5385, 3.5619) -> (-6.2857, 3.5619)
  line L179 (-6.2857, 3.5619) -> (-6.2857, 2.0611)
  line L180 (-6.2679, 3.8115) -> (-6.5548, 3.8115)
  line L181 (-6.5548, 3.8115) -> (-6.5548, 4.0741)
  line L182 (-6.5548, 4.0741) -> (-6.2679, 4.0741)
  line L183 (-6.2679, 4.0741) -> (-6.2679, 3.8115)
  spline S181 degree 2 poles (-4.6569, 2.8358) (-4.6569, 2.4679) (-5.0134, 2.019) (-5.2825, 2.019) knots 0 0 0 1 2 2 2
  spline S182 degree 2 poles (-5.2825, 2.019) (-5.404, 2.019) (-5.5774, 2.0789) (-5.6617, 2.1308) knots 0 0 0 1 2 2 2
  line L184 (-5.6617, 2.1308) -> (-5.6779, 2.0611)
  line L185 (-5.6779, 2.0611) -> (-5.9146, 2.0611)
  line L186 (-5.9146, 2.0611) -> (-5.9146, 4.1503)
  line L187 (-5.9146, 4.1503) -> (-5.6617, 4.1503)
  line L188 (-5.6617, 4.1503) -> (-5.6617, 3.4047)
  spline S183 degree 2 poles (-5.6617, 3.4047) (-5.5661, 3.4906) (-5.3441, 3.6041) (-5.203, 3.6041) knots 0 0 0 1 2 2 2
  spline S184 degree 2 poles (-5.203, 3.6041) (-4.9486, 3.6041) (-4.6569, 3.1973) (-4.6569, 2.8358) knots 0 0 0 1 2 2 2
  spline S185 degree 2 poles (-4.9178, 2.8164) (-4.9178, 3.0854) (-5.0815, 3.3642) (-5.263, 3.3642) knots 0 0 0 1 2 2 2
  spline S186 degree 2 poles (-5.263, 3.3642) (-5.3651, 3.3642) (-5.5758, 3.267) (-5.6617, 3.1924) knots 0 0 0 1 2 2 2
  line L189 (-5.6617, 3.1924) -> (-5.6617, 2.3318)
  spline S187 degree 2 poles (-5.6617, 2.3318) (-5.5661, 2.2848) (-5.4186, 2.2459) (-5.3311, 2.2459) knots 0 0 0 1 2 2 2
  spline S188 degree 2 poles (-5.3311, 2.2459) (-5.1382, 2.2459) (-4.9178, 2.5198) (-4.9178, 2.8164) knots 0 0 0 1 2 2 2
  line L190 (-3.2274, 2.0611) -> (-3.4802, 2.0611)
  line L191 (-3.4802, 2.0611) -> (-3.4802, 2.2264)
  spline S189 degree 2 poles (-3.4802, 2.2264) (-3.5969, 2.1243) (-3.806, 2.019) (-3.9356, 2.019) knots 0 0 0 1 2 2 2
  spline S190 degree 2 poles (-3.9356, 2.019) (-4.0329, 2.019) (-4.2063, 2.0838) (-4.2695, 2.1535) knots 0 0 0 1 2 2 2
  spline S191 degree 2 poles (-4.2695, 2.1535) (-4.3343, 2.2232) (-4.4056, 2.4355) (-4.4056, 2.5879) knots 0 0 0 1 2 2 2
  line L192 (-4.4056, 2.5879) -> (-4.4056, 3.5619)
  line L193 (-4.4056, 3.5619) -> (-4.1528, 3.5619)
  line L194 (-4.1528, 3.5619) -> (-4.1528, 2.7062)
  spline S192 degree 2 poles (-4.1528, 2.7062) (-4.1528, 2.5862) (-4.135, 2.429) (-4.1042, 2.3707) knots 0 0 0 1 2 2 2
  spline S193 degree 2 poles (-4.1042, 2.3707) (-4.0734, 2.3123) (-3.968, 2.2589) (-3.8692, 2.2589) knots 0 0 0 1 2 2 2
  spline S194 degree 2 poles (-3.8692, 2.2589) (-3.7768, 2.2589) (-3.5677, 2.3642) (-3.4802, 2.4404) knots 0 0 0 1 2 2 2
  line L195 (-3.4802, 2.4404) -> (-3.4802, 3.5619)
  line L196 (-3.4802, 3.5619) -> (-3.2274, 3.5619)
  line L197 (-3.2274, 3.5619) -> (-3.2274, 2.0611)
  spline S195 degree 2 poles (-2.2646, 2.0271) (-2.4202, 2.0271) (-2.6779, 2.1227) (-2.7703, 2.22) knots 0 0 0 1 2 2 2
  spline S196 degree 2 poles (-2.7703, 2.22) (-2.8627, 2.3156) (-2.9648, 2.6106) (-2.9648, 2.8083) knots 0 0 0 1 2 2 2
  spline S197 degree 2 poles (-2.9648, 2.8083) (-2.9648, 3.006) (-2.8595, 3.2945) (-2.7703, 3.3918) knots 0 0 0 1 2 2 2
  spline S198 degree 2 poles (-2.7703, 3.3918) (-2.6812, 3.4906) (-2.417, 3.596) (-2.2646, 3.596) knots 0 0 0 1 2 2 2
  spline S199 degree 2 poles (-2.2646, 3.596) (-2.1415, 3.596) (-1.9113, 3.5263) (-1.8222, 3.4809) knots 0 0 0 1 2 2 2
  line L198 (-1.8222, 3.4809) -> (-1.8222, 3.1973)
  line L199 (-1.8222, 3.1973) -> (-1.8368, 3.1973)
  spline S200 degree 2 poles (-1.8368, 3.1973) (-1.8643, 3.22) (-1.9486, 3.2783) (-2.0086, 3.3091) knots 0 0 0 1 2 2 2
  spline S201 degree 2 poles (-2.0086, 3.3091) (-2.062, 3.335) (-2.2047, 3.3755) (-2.2695, 3.3755) knots 0 0 0 1 2 2 2
  spline S202 degree 2 poles (-2.2695, 3.3755) (-2.4656, 3.3755) (-2.7039, 3.0789) (-2.7039, 2.8083) knots 0 0 0 1 2 2 2
  spline S203 degree 2 poles (-2.7039, 2.8083) (-2.7039, 2.5441) (-2.4737, 2.2475) (-2.2695, 2.2475) knots 0 0 0 1 2 2 2
  spline S204 degree 2 poles (-2.2695, 2.2475) (-2.1463, 2.2475) (-1.9227, 2.3496) (-1.8368, 2.429) knots 0 0 0 1 2 2 2
  line L200 (-1.8368, 2.429) -> (-1.8222, 2.429)
  line L201 (-1.8222, 2.429) -> (-1.8222, 2.1454)
  spline S205 degree 2 poles (-1.8222, 2.1454) (-1.8595, 2.1276) (-1.9729, 2.0773) (-2.0183, 2.066) knots 0 0 0 1 2 2 2
  spline S206 degree 2 poles (-2.0183, 2.066) (-2.0831, 2.0465) (-2.1852, 2.0271) (-2.2646, 2.0271) knots 0 0 0 1 2 2 2
  spline S207 degree 2 poles (-0.9405, 2.0271) (-1.3003, 2.0271) (-1.6958, 2.4307) (-1.6958, 2.8034) knots 0 0 0 1 2 2 2
  spline S208 degree 2 poles (-1.6958, 2.8034) (-1.6958, 3.1697) (-1.3116, 3.6041) (-1.0021, 3.6041) knots 0 0 0 1 2 2 2
  spline S209 degree 2 poles (-1.0021, 3.6041) (-0.8627, 3.6041) (-0.6471, 3.523) (-0.5677, 3.4371) knots 0 0 0 1 2 2 2
  spline S210 degree 2 poles (-0.5677, 3.4371) (-0.4867, 3.3512) (-0.4008, 3.1033) (-0.4008, 2.9234) knots 0 0 0 1 2 2 2
  line L202 (-0.4008, 2.9234) -> (-0.4008, 2.7856)
  line L203 (-0.4008, 2.7856) -> (-1.4397, 2.7856)
  spline S211 degree 2 poles (-1.4397, 2.7856) (-1.4397, 2.5247) (-1.1771, 2.2475) (-0.9437, 2.2475) knots 0 0 0 1 2 2 2
  spline S212 degree 2 poles (-0.9437, 2.2475) (-0.8611, 2.2475) (-0.7006, 2.2848) (-0.6358, 2.314) knots 0 0 0 1 2 2 2
  spline S213 degree 2 poles (-0.6358, 2.314) (-0.5677, 2.3464) (-0.4737, 2.4031) (-0.4429, 2.429) knots 0 0 0 1 2 2 2
  line L204 (-0.4429, 2.429) -> (-0.4283, 2.429)
  line L205 (-0.4283, 2.429) -> (-0.4283, 2.1535)
  spline S214 degree 2 poles (-0.4283, 2.1535) (-0.4721, 2.1357) (-0.605, 2.0838) (-0.6569, 2.0692) knots 0 0 0 1 2 2 2
  spline S215 degree 2 poles (-0.6569, 2.0692) (-0.7298, 2.0482) (-0.8497, 2.0271) (-0.9405, 2.0271) knots 0 0 0 1 2 2 2
  spline S216 degree 2 poles (-0.6471, 2.9785) (-0.6504, 3.0806) (-0.6925, 3.2297) (-0.733, 3.2799) knots 0 0 0 1 2 2 2
  spline S217 degree 2 poles (-0.733, 3.2799) (-0.7768, 3.3366) (-0.9146, 3.3966) (-1.0167, 3.3966) knots 0 0 0 1 2 2 2
  spline S218 degree 2 poles (-1.0167, 3.3966) (-1.1171, 3.3966) (-1.2582, 3.3366) (-1.3165, 3.2783) knots 0 0 0 1 2 2 2
  spline S219 degree 2 poles (-1.3165, 3.2783) (-1.3732, 3.2183) (-1.4316, 3.0741) (-1.4397, 2.9785) knots 0 0 0 1 2 2 2
  line L206 (-1.4397, 2.9785) -> (-0.6471, 2.9785)
  point P0 (0, 0)
  constraints: 2 other
emboss "Reliéf1" sketch "Náčrt6" operation add depth 0.01 direction (0, 0, -1)